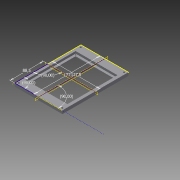
# Autodesk Inventor part: transillum_diffusor_partA_v3
Saved by Autodesk Inventor 2015 (Build 190159000, 159)
## iProperties
Created: 2022-05-26
Part Number: transillum_diffusor_partA_v3
Material: Genérico
Document SubType Name: Modeling
Designer: Zuloaga
Density: 1 g/cm^3
Appearance: Valor por defecto
Author: Zuloaga
Autodesk Inventor part; units mm, degrees
ref_plane "YZ Plane" through (0, 0, 0) normal (1, 0, 0) x (0, 1, 0)
ref_plane "XZ Plane" through (0, 0, 0) normal (0, 1, 0) x (-1, 0, 0)
ref_plane "XY Plane" through (0, 0, 0) normal (0, 0, 1) x (1, 0, 0)
sketch "Boceto1" plane through (0, 0, 0) normal (0, 0, 1) x (1, 0, 0)
  line L0 (0, 0) -> (127.5, 0)
  line L1 (127.5, 0) -> (127.5, 177)
  line L2 (127.5, 177) -> (0, 177)
  line L3 (0, 177) -> (0, 0)
  dimension "d32" = 127.5
  dimension "d33" = 177
  constraints: 8 end point, 2 parallel, 1 horizontal, 1 perpendicular
  measures "d32" distance of L2.end L1.end
  measures "d33" distance of L1.end L0.end
extrude "Extrusión1" add sketch "Boceto1" along normal blind 2.5
sketch "Boceto2" plane through (0, 0, 2.5) normal (0, 0, 1) x (1, 0, 0)
  line L0 (127.5, 0) -> (127.5, 27.5)
  line L1 (127.5, 0) -> (127.5, 177) projected
  line L2 (127.5, 0) -> (155, 0) construction
  line L3 (127.5, 27.5) -> (113.75, 27.5)
  line L4 (0, 0) -> (127.5, 0) projected
  line L5 (113.75, 27.5) -> (13.75, 27.5)
  line L6 (13.75, 27.5) -> (13.75, 149.5)
  line L7 (13.75, 149.5) -> (113.75, 149.5)
  line L8 (113.75, 149.5) -> (113.75, 27.5)
  dimension "d36" = 27.5
  dimension "d37" = 90
  dimension "d38" = 13.75
  dimension "d39" = 90
  dimension "d40" = 100
  dimension "d41" = 122
  constraints: 14 end point, 3 parallel, 2 horizontal, 2 perpendicular, 1 collinear
  measures "d36" distance of L0.start L0.end
  measures "d37" angle of L2 L0
  measures "d38" distance of L0.end L3.end
  measures "d39" angle of L3 L0
  measures "d40" distance of L6.end L7.end
  measures "d41" distance of L5.end L6.end
extrude "Extrusión2" cut sketch "Boceto2" against normal blind 2.5
sketch "Boceto3" plane through (0, 0, 2.5) normal (0, 0, 1) x (1, 0, 0)
  line L0 (13.75, 149.5) -> (7.75, 149.5)
  line L1 (7.75, 149.5) -> (7.75, 155.5)
  line L2 (113.75, 27.5) -> (113.75, 21.5)
  line L3 (113.75, 27.5) -> (119.75, 27.5) construction
  line L4 (113.75, 21.5) -> (119.75, 21.5)
  line L5 (7.75, 155.5) -> (119.75, 155.5)
  line L6 (119.75, 155.5) -> (119.75, 21.5)
  line L7 (119.75, 21.5) -> (7.75, 21.5)
  line L8 (7.75, 21.5) -> (7.75, 155.5)
  line L9 (0, 177) -> (127.5, 177)
  line L10 (127.5, 177) -> (127.5, 0)
  line L11 (127.5, 0) -> (0, 0)
  line L12 (0, 0) -> (0, 177)
  dimension "d44" = 6
  dimension "d45" = 6
  dimension "d46" = 90
  dimension "d47" = 6
  dimension "d48" = 90
  dimension "d49" = 6
  dimension "d50" = 90
  constraints: 26 end point, 5 perpendicular, 4 horizontal, 4 parallel, 1 vertical
  measures "d44" distance of L0.start L0.end
  measures "d45" distance of L0.end L1.end
  measures "d46" angle of L0 L1
  measures "d47" distance of L2.start L2.end
  measures "d48" angle of L2 L3
  measures "d49" distance of L2.end L4.end
  measures "d50" angle of L4 L2
extrude "Extrusión3" add sketch "Boceto3" along normal blind 6
sketch "Boceto6" plane through (0, 0, 8.5) normal (0, 0, 1) x (1, 0, 0)
  line L0 (0, 0) -> (0, 88.5)
  line L1 (0, 177) -> (0, 0) projected
  line L2 (0, 0) -> (88.5, 0) construction
  line L3 (0, 88.5) -> (127.5, 88.5)
  dimension "d73" = 88.5
  dimension "d74" = 90
  dimension "d75" = 127.5
  dimension "d76" = 90
  constraints: 6 end point, 2 perpendicular, 1 collinear, 1 horizontal
  measures "d73" distance of L0.start L0.end
  measures "d74" angle of L2 L0
  measures "d75" distance of L0.end L3.end
  measures "d76" angle of L0 L3
ref_plane "Plano de trabajo1" through (0, 88.5, 8.5) normal (0, -1, 0) x (1, 0, 0)
sketch "Boceto7" plane through (0, 0, 8.5) normal (0, 0, 1) x (1, 0, 0)
  line L0 (0, 0) -> (63.75, 0)
  line L1 (0, 0) -> (127.5, 0) projected
  line L2 (63.75, 0) -> (63.75, 177)
  line L3 (127.5, 177) -> (0, 177) projected
  line L4 (63.75, 0) -> (240.75, 0) construction
  dimension "d78" = 177
  dimension "d79" = 90
  constraints: 6 end point, 2 perpendicular, 1 horizontal, 1 midpoint
  measures "d78" distance of L0.end L2.end
  measures "d79" angle of L4 L2
ref_plane "Plano de trabajo2" through (63.75, 0, 8.5) normal (1, 0, 0) x (0, 1, 0)
sketch "Boceto8" plane through (0, 0, 2.5) normal (0, 0, 1) x (1, 0, 0)
  line L0 (13.75, 27.5) -> (7.75, 27.5)
  line L1 (7.75, 27.5) -> (7.75, 21.5)
  line L2 (7.75, 21.5) -> (13.75, 21.5)
  line L3 (13.75, 21.5) -> (13.75, 27.5)
  line L4 (13.75, 21.5) -> (7.75, 27.5)
  line L5 (13.75, 27.5) -> (7.75, 21.5)
  circle A0 centre (10.75, 24.5) radius 1.6
  point P0 (0, 0)
  dimension "d81" = 6
  dimension "d82" = 6
  dimension "d83" = 3.2
  constraints: 12 end point, 2 parallel, 1 centre point, 1 horizontal, 1 midpoint, 1 perpendicular
  measures "d81" distance of L2.end L1.end
  measures "d82" distance of L1.end L0.end
  measures "d83" diameter of A0
extrude "Extrusión4" cut sketch "Boceto8" against normal blind 4 contours A0 L4 L5 | L5 L4 A0 | L4 L5 A0 | A0 L5 L4
mirror "Simetría1" about plane through (63.75, 0, 8.5) normal (1, 0, 0) of "Extrusión4"
mirror "Simetría2" about plane through (0, 88.5, 8.5) normal (0, -1, 0) of "Extrusión4", "Simetría1"
sketch "Boceto9" plane through (0, 0, 8.5) normal (0, 0, 1) x (1, 0, 0)
  line L0 (0, 177) -> (11.5, 177)
  line L1 (11.5, 177) -> (11.5, 165.5)
  line L2 (11.5, 165.5) -> (0, 165.5)
  line L3 (0, 165.5) -> (0, 177)
  line L4 (0, 177) -> (11.5, 165.5)
  line L5 (0, 165.5) -> (11.5, 177)
  circle A0 centre (5.75, 171.25) radius 2.1
  point P0 (0, 0)
  dimension "d86" = 11.5
  dimension "d87" = 11.5
  dimension "d88" = 4.2
  constraints: 12 end point, 2 parallel, 1 centre point, 1 horizontal, 1 midpoint, 1 perpendicular
  measures "d86" distance of L1.end L2.end
  measures "d87" distance of L0.end L1.end
  measures "d88" diameter of A0
extrude "Extrusión5" cut sketch "Boceto9" against normal blind 10 contours A0 L5 L4 | L4 L5 A0 | A0 L4 L5 | L5 L4 A0
mirror "Simetría3" about plane through (63.75, 0, 8.5) normal (1, 0, 0) of "Extrusión5"
mirror "Simetría4" about plane through (0, 88.5, 8.5) normal (0, -1, 0) of "Extrusión5", "Simetría3"
